Heatstand (Autodesk Fusion 360 design; units mm, degrees)
Autodesk Fusion 360 part; units mm, degrees
note: some values were not read from the file. Set by a fixed rule: which sketch regions a step uses.
sketch "Sketch1" plane through (0, 0, 0) normal (0, 0, 1) x (1, 0, 0)
  circle A0 centre (0, 0) radius 14.5
  line L0 (19.5, -19.5) -> (34.5, -19.5)
  line L1 (34.5, -19.5) -> (34.5, 19.5)
  line L2 (34.5, 19.5) -> (19.5, 19.5)
  line L3 (19.5, 19.5) -> (19.5, -19.5)
  line L4 (-19.5, 19.5) -> (39.5, 19.5)
  line L5 (39.5, 19.5) -> (39.5, -19.5)
  line L6 (39.5, -19.5) -> (-19.5, -19.5)
  line L7 (-19.5, -19.5) -> (-19.5, 19.5)
  dimension "d1" = 29
  dimension "d2" = 15
  dimension "d3" = 19.5
  dimension "d6" = 19.5
  dimension "d7" = 19.5
  dimension "d8" = 19.5
  dimension "d9" = 5
  constraint coincident A0.centre origin
  constraint horizontal L0
  constraint vertical L1
  constraint horizontal L2
  constraint vertical L3
  constraint horizontal L4
  constraint vertical L5
  constraint horizontal L6
  constraint vertical L7
  constraint coincident L1.end L4
  constraint coincident L0.end L6
  measures "d1" diameter of A0
  measures "d2" distance of L0.start L0.end
  measures "d3" distance of A0.centre L3
  measures "d6" distance of A0.centre L4
  measures "d7" distance of A0.centre L7
  measures "d8" distance of A0.centre L6
  measures "d9" distance of L1 L5
extrude "Extrude1" add sketch "Sketch1" against normal blind 10
extrude "Extrude2" add sketch "Sketch1" against normal blind 110 contours L3 L4 L6 L7 | L1 L4 L5 L6
extrude "Extrude3" add sketch "Sketch1" against normal blind 125 contours L3 L4 L6 L7
fillet "Fillet1" radius 19.5 2 edges at (-19.5, 19.5, -62.5) (-19.5, -19.5, -62.5)
fillet "Fillet2" radius 7.5 1 edges at (39.5, 0, 0)
sketch "Sketch2" plane through (39.5, 0, 0) normal (1, 0, 0) x (0, 1, 0)
  line L0 (19.5, -7.5) -> (-19.5, -7.5)
  line L1 (-19.5, -7.5) -> (-19.5, -110)
  line L2 (-19.5, -110) -> (19.5, -110)
  line L3 (19.5, -110) -> (19.5, -7.5)
  circle A0 centre (0, -27.5) radius 1.5
  line L4 (19.5, 0) -> (-19.5, 0)
  circle A1 centre (0, -90) radius 1.5
  circle A2 centre (0, -58.75) radius 1.5
  dimension "d22" = 3
  dimension "d25" = 3
  dimension "d26" = 20
  dimension "d27" = 3
  dimension "d29" = 20
  dimension "d30" = 51.25
  measures "d22" diameter of A0
  measures "d25" diameter of A1
  measures "d26" distance of L2 A1.centre
  measures "d27" diameter of A2
  measures "d29" distance of L0 A0.centre
  measures "d30" distance of L0 A2.centre
extrude "Extrude4" cut sketch "Sketch2" against normal blind 5 contours A0 | A1 | A2
sketch "Sketch3" plane through (19.5, 0, 0) normal (1, 0, 0) x (0, 1, 0)
  line L0 (19.5, -10) -> (-19.5, -10)
  line L1 (-19.5, -10) -> (-19.5, -125)
  line L2 (-19.5, -125) -> (19.5, -125)
  line L3 (19.5, -125) -> (19.5, -10)
  circle A0 centre (0, -20) radius 4
  circle A1 centre (0, -105) radius 4
  circle A2 centre (0, -62.5) radius 4
  line L4 (-19.5, 0) -> (19.5, 0)
  line L5 (0, 0) -> (0, -125)
  circle A3 centre (0, -20) radius 1.5
  circle A4 centre (0, -62.5) radius 1.5
  circle A5 centre (0, -105) radius 1.5
  circle A6 centre (0, -41.25) radius 1.5
  circle A7 centre (0, -83.75) radius 1.5
  line L6 (0, -20) -> (0, -62.5)
  line L7 (0, -105) -> (0, -62.5)
  dimension "d34" = 8
  dimension "d35" = 8
  dimension "d36" = 8
  dimension "d37" = 20
  dimension "d38" = 20
  dimension "d42" = 3
  dimension "d43" = 3
  dimension "d44" = 3
  dimension "d47" = 3
  dimension "d48" = 3
  constraint coincident L5.start origin
  constraint midpoint L2 L5.end
  constraint midpoint A2.centre L5
  constraint concentric A0 A3
  constraint concentric A2 A4
  constraint concentric A1 A5
  constraint coincident L5 A6.centre
  constraint coincident L5 A7.centre
  constraint coincident A0.centre A3.centre
  constraint coincident A2.centre A4.centre
  constraint parallel L5 L6
  constraint coincident A1.centre A5.centre
  constraint parallel L5 L7
  constraint midpoint A6.centre L6
  constraint midpoint A7.centre L7
  measures "d34" diameter of A0
  measures "d35" diameter of A1
  measures "d36" diameter of A2
  measures "d37" distance of A0.centre L4
  measures "d38" distance of L2 A1.centre
  measures "d42" diameter of A3
  measures "d43" diameter of A4
  measures "d44" diameter of A5
  measures "d47" diameter of A6
  measures "d48" diameter of A7
extrude "Extrude5" cut sketch "Sketch3" against normal blind 20 from surface at -29 contours A0 L5 A3 L6 | A0 L5 A3 L6 | L5 A3 L6 | L5 A3 L6 | A1 L5 A5 L7 | A1 L5 A5 L7 | L5 A5 L7 | L5 A5 L7 | A2 L5 A4 L6 L7 | A2 L5 A4 L6 L7 | L5 A4 L6 L7 | L5 A4 L6 L7
extrude "Extrude6" cut sketch "Sketch3" against normal blind 100 contours L5 A3 L6 | L5 A3 L6 | L5 A5 L7 | L5 A5 L7 | L5 A4 L6 L7 | L5 A4 L6 L7
extrude "Extrude7" cut sketch "Sketch3" against normal blind 40 from surface at -10 contours L5 A6 L6 | L5 A6 L6 | L5 A7 L7 | L5 A7 L7
chamfer "Chamfer1" distance 1 angle 45 8 edges at (-19.4422, -1.5, -41.25) (-19.4422, -1.5, -83.75) (14.4222, -1.5, -20) (14.4222, -1.5, -62.5) (14.4222, -1.5, -105) (39.5, -1.3985, -26.9576) (39.5, -1.3985, -58.2076) (39.5, -1.3985, -89.4576)
equation "d1 = diameter_stick"
equation "d3 = ( diameter_stick / 2 ) + thickness"
equation "diameter_stick = 29 mm"
equation "thickness = 5 mm"
equation "d6 = ( diameter_stick / 2 ) + thickness"
equation "d7 = ( diameter_stick / 2 ) + thickness"
equation "d8 = ( diameter_stick / 2 ) + thickness"
equation "d9 = thickness"
equation "d10 = -( thickness * 2 )"
equation "d12 = -( ( thickness * 2 ) + height_inner )"
equation "height_inner = 100 mm"
equation "height_outer = 115 mm"
equation "d16 = -( ( thickness * 2 ) + height_outer )"
equation "d19 = ( diameter_stick / 2 ) + thickness"
equation "d22 = screw_hole"
equation "screw_hole = 3 mm"
equation "d25 = screw_hole"
equation "d27 = screw_hole"
equation "d30 = ( 102.5 / 2 ) * 1 mm"
equation "d31 = -thickness"
equation "driver_hole = 8 mm"
equation "d34 = driver_hole"
equation "d35 = driver_hole"
equation "d36 = driver_hole"
equation "d39 = -( thickness + diameter_stick - 5 mm )"
equation "d42 = screw_hole"
equation "d43 = screw_hole"
equation "d44 = screw_hole"
equation "d47 = screw_hole"
equation "d48 = screw_hole"
equation "screw_chamfer = 1 mm"
equation "d50 = screw_chamfer"
equation "d52 = -( thickness * 2 )"
